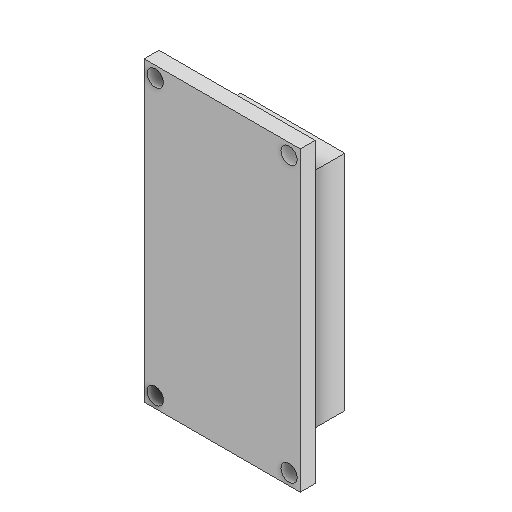
# Autodesk Inventor part: 7_Seg_Display_TM1637
Saved by Autodesk Inventor 2026.2 (Build 302298010, 298A)
## iProperties
Created: 2026-03-17
Part Number: 7_Seg_Display_TM1637
Material: Generic
Document SubType Name: Modeling
Designer: vckot
Density: 1 g/cm^3
Appearance: Default
Author: vckot
Autodesk Inventor part; units mm, degrees
ref_plane "YZ Plane" through (0, 0, 0) normal (1, 0, 0) x (0, 1, 0)
ref_plane "XZ Plane" through (0, 0, 0) normal (0, 1, 0) x (-1, 0, 0)
ref_plane "XY Plane" through (0, 0, 0) normal (0, 0, 1) x (1, 0, 0)
sketch "Sketch1" plane through (0, 0, 0) normal (0, 1, 0) x (-1, 0, 0)
  line L0 (-10.5, 20) -> (10.5, 20)
  line L1 (10.5, 20) -> (10.5, -20)
  line L2 (10.5, -20) -> (-10.5, -20)
  line L3 (-10.5, -20) -> (-10.5, 20)
  line L4 (-10.5, 20) -> (10.5, -20) construction
  line L5 (10.5, 20) -> (-10.5, -20) construction
  point P0 (0, 0)
  dimension "d0" = 40
  dimension "d1" = 21
  constraints: 12 end point, 2 midpoint, 2 parallel, 1 horizontal, 1 perpendicular
  measures "d0" distance of L0.end L1.end
  measures "d1" distance of L1.end L2.end
extrude "Extrusion1" add sketch "Sketch1" along normal blind 2
sketch "Sketch2" plane through (0, 2, 0) normal (0, 1, 0) x (1, 0, 0)
  line L0 (-10.5, 20) -> (-10.5, -20) projected
  line L1 (-10.5, -20) -> (10.5, -20) projected
  line L2 (10.5, -20) -> (10.5, 20) projected
  line L3 (10.5, 20) -> (-10.5, 20) projected
  point P0 (0, 0)
  point P1 (-9, -18.5)
  point P2 (-9, 18.5)
  point P3 (9, 18.5)
  point P4 (9, -18.5)
  dimension "d4" = 1.5
  dimension "d5" = 1.5
  dimension "d6" = 1.5
  dimension "d7" = 1.5
  dimension "d20" = 18
  dimension "d21" = 18
  dimension "d22" = 37
  constraints: 2 horizontal alignment, 2 vertical alignment
  measures "d4" distance from line of L0 point (-9, -18.5)
  measures "d5" distance from line of L1 point (-9, -18.5)
  measures "d6" distance from line of L2 point (9, -18.5)
  measures "d7" distance from line of L3 point (-9, 18.5)
  measures "d20" distance of point (9, 18.5) point (-9, 18.5)
  measures "d21" distance of point (9, -18.5) point (-9, -18.5)
  measures "d22" distance of point (-9, 18.5) point (-9, -18.5)
hole "Hole1" at (-9, 2, 18.5) at (-9, 2, -18.5) at (9, 2, -18.5) at (9, 2, 18.5) direction (0, -1, 0) diameter 2.2 end through all
sketch "Sketch3" plane through (0, 2, 0) normal (0, 1, 0) x (1, 0, 0)
  line L0 (7.5, -13.5) -> (-6.5, -13.5)
  line L1 (-6.5, -13.5) -> (-6.5, 16.5)
  line L2 (-6.5, 16.5) -> (7.5, 16.5)
  line L3 (7.5, 16.5) -> (7.5, -13.5)
  line L4 (7.5, -13.5) -> (-6.5, 16.5) construction
  line L5 (-6.5, -13.5) -> (7.5, 16.5) construction
  line L6 (-10.5, -20) -> (10.5, -20) projected
  line L7 (-10.5, 20) -> (-10.5, -20) projected
  line L8 (10.5, 20) -> (-10.5, 20) projected
  point P0 (0, 0)
  point P1 (0.5, 1.5)
  point P2 (0, -20)
  dimension "d15" = 6.5
  dimension "d16" = 30
  dimension "d17" = 14
  dimension "d18" = 4
  dimension "d19" = 3.5
  constraints: 12 end point, 3 midpoint, 2 parallel, 1 horizontal, 1 perpendicular
  measures "d15" distance from line of point (0, -20) L0
  measures "d16" distance of L0.end L1.end
  measures "d17" distance of L1.end L2.end
  measures "d18" distance between parallel lines of L7 L1
  measures "d19" distance between parallel lines of L8 L2
extrude "Extrusion2" add sketch "Sketch3" along normal blind 7
sketch "Sketch4" plane through (0, 9, 0) normal (0, 1, 0) x (1, 0, 0)
  line L0 (-6.5, -13.5) -> (7.5, -13.5) projected
  line L1 (10.5, -20) -> (10.5, 20) projected
  line L2 (-6.5, 16.5) -> (-6.5, -13.5) projected
  line L3 (-0.449, -7.3714) -> (-0.0305, -6.9347)
  line L4 (-0.0305, -6.9347) -> (0.3941, -7.3714)
  line L5 (0.3941, -7.3714) -> (0.3941, -10.3494)
  line L6 (0.3941, -10.3494) -> (-0.0305, -10.774)
  line L7 (-0.0305, -10.774) -> (-0.449, -10.3494)
  line L8 (-0.449, -10.3494) -> (-0.449, -7.3714)
  line L9 (-0.5096, -11.2532) -> (-4.0275, -11.2532)
  line L10 (-4.0275, -11.2532) -> (-3.1723, -10.398)
  line L11 (-3.1723, -10.398) -> (-0.728, -10.398)
  line L12 (-0.728, -10.398) -> (-0.1882, -10.9317)
  line L13 (-0.1882, -10.9317) -> (-0.5096, -11.2532)
  line L14 (0.6731, -10.398) -> (3.1174, -10.398)
  line L15 (3.1174, -10.398) -> (3.9725, -11.2532)
  line L16 (3.9725, -11.2532) -> (0.4669, -11.2532)
  line L17 (0.4669, -11.2532) -> (0.1333, -10.9317)
  line L18 (0.1333, -10.9317) -> (0.6731, -10.398)
  line L19 (-0.7219, -7.3108) -> (-3.1662, -7.3108)
  line L20 (-3.1662, -7.3108) -> (-4.0275, -6.4677)
  line L21 (-4.0275, -6.4677) -> (-0.5036, -6.4677)
  line L22 (-0.5036, -6.4677) -> (-0.1882, -6.777)
  line L23 (-0.1882, -6.777) -> (-0.7219, -7.3108)
  line L24 (0.4669, -6.4677) -> (3.9725, -6.4677)
  line L25 (3.9725, -6.4677) -> (3.1174, -7.3108)
  line L26 (3.1174, -7.3108) -> (0.6731, -7.3108)
  line L27 (0.6731, -7.3108) -> (0.1333, -6.777)
  line L28 (0.1333, -6.777) -> (0.4669, -6.4677)
  line L29 (-0.449, -1.2092) -> (-0.0305, -0.7725)
  line L30 (-0.0305, -0.7725) -> (0.3941, -1.2092)
  line L31 (0.3941, -1.2092) -> (0.3941, -4.1872)
  line L32 (0.3941, -4.1872) -> (-0.0305, -4.6118)
  line L33 (-0.0305, -4.6118) -> (-0.449, -4.1872)
  line L34 (-0.449, -4.1872) -> (-0.449, -1.2092)
  line L35 (-0.5096, -5.0909) -> (-4.0275, -5.0909)
  line L36 (-4.0275, -5.0909) -> (-3.1723, -4.2357)
  line L37 (-3.1723, -4.2357) -> (-0.728, -4.2357)
  line L38 (-0.728, -4.2357) -> (-0.1882, -4.7695)
  line L39 (-0.1882, -4.7695) -> (-0.5096, -5.0909)
  line L40 (0.6731, -4.2357) -> (3.1174, -4.2357)
  line L41 (3.1174, -4.2357) -> (3.9725, -5.0909)
  line L42 (3.9725, -5.0909) -> (0.4669, -5.0909)
  line L43 (0.4669, -5.0909) -> (0.1333, -4.7695)
  line L44 (0.1333, -4.7695) -> (0.6731, -4.2357)
  line L45 (-0.7219, -1.1485) -> (-3.1662, -1.1485)
  line L46 (-3.1662, -1.1485) -> (-4.0275, -0.3055)
  line L47 (-4.0275, -0.3055) -> (-0.5036, -0.3055)
  line L48 (-0.5036, -0.3055) -> (-0.1882, -0.6148)
  line L49 (-0.1882, -0.6148) -> (-0.7219, -1.1485)
  line L50 (0.4669, -0.3055) -> (3.9725, -0.3055)
  line L51 (3.9725, -0.3055) -> (3.1174, -1.1485)
  line L52 (3.1174, -1.1485) -> (0.6731, -1.1485)
  line L53 (0.6731, -1.1485) -> (0.1333, -0.6148)
  line L54 (0.1333, -0.6148) -> (0.4669, -0.3055)
  line L55 (-1.8319, 1.3321) -> (-2.687, 1.3321)
  line L56 (-2.687, 1.3321) -> (-2.687, 2.1873)
  line L57 (-2.687, 2.1873) -> (-1.8319, 2.1873)
  line L58 (-1.8319, 2.1873) -> (-1.8319, 1.3321)
  line L59 (3.9725, 1.3321) -> (3.1174, 1.3321)
  line L60 (3.1174, 1.3321) -> (3.1174, 2.1873)
  line L61 (3.1174, 2.1873) -> (3.9725, 2.1873)
  line L62 (3.9725, 2.1873) -> (3.9725, 1.3321)
  line L63 (-4.0275, 8.4527) -> (-3.1723, 7.6035)
  line L64 (-3.1723, 7.6035) -> (-3.1723, 4.8257)
  line L65 (-3.1723, 4.8257) -> (-4.0275, 3.9826)
  line L66 (-4.0275, 3.9826) -> (-4.0275, 8.4527)
  line L67 (0.6731, 4.6801) -> (3.1174, 4.6801)
  line L68 (3.1174, 4.6801) -> (3.9725, 3.8249)
  line L69 (3.9725, 3.8249) -> (0.4669, 3.8249)
  line L70 (0.4669, 3.8249) -> (0.1333, 4.1464)
  line L71 (0.1333, 4.1464) -> (0.6731, 4.6801)
  line L72 (0.4669, 8.6104) -> (3.9725, 8.6104)
  line L73 (3.9725, 8.6104) -> (3.1174, 7.7673)
  line L74 (3.1174, 7.7673) -> (0.6731, 7.7673)
  line L75 (0.6731, 7.7673) -> (0.1333, 8.301)
  line L76 (0.1333, 8.301) -> (0.4669, 8.6104)
  line L77 (-0.5096, 3.8249) -> (-3.8698, 3.8249)
  line L78 (-3.8698, 3.8249) -> (-3.0085, 4.6801)
  line L79 (-3.0085, 4.6801) -> (-0.728, 4.6801)
  line L80 (-0.728, 4.6801) -> (-0.1882, 4.1464)
  line L81 (-0.1882, 4.1464) -> (-0.5096, 3.8249)
  line L82 (-0.7219, 7.7673) -> (-3.0085, 7.7673)
  line L83 (-3.0085, 7.7673) -> (-3.8637, 8.6104)
  line L84 (-3.8637, 8.6104) -> (-0.5036, 8.6104)
  line L85 (-0.5036, 8.6104) -> (-0.1882, 8.301)
  line L86 (-0.1882, 8.301) -> (-0.7219, 7.7673)
  line L87 (-2.5294, 5.7901) -> (-2.9539, 6.2146)
  line L88 (-2.9539, 6.2146) -> (-2.5294, 6.6452)
  line L89 (-2.5294, 6.6452) -> (-0.6249, 6.6452)
  line L90 (-0.6249, 6.6452) -> (-0.1882, 6.2146)
  line L91 (-0.1882, 6.2146) -> (-0.6249, 5.7901)
  line L92 (-0.6249, 5.7901) -> (-2.5294, 5.7901)
  line L93 (-4.0275, 14.6149) -> (-3.1723, 13.7658)
  line L94 (-3.1723, 13.7658) -> (-3.1723, 10.9879)
  line L95 (-3.1723, 10.9879) -> (-4.0275, 10.1449)
  line L96 (-4.0275, 10.1449) -> (-4.0275, 14.6149)
  line L97 (0.6731, 10.8424) -> (3.1174, 10.8424)
  line L98 (3.1174, 10.8424) -> (3.9725, 9.9872)
  line L99 (3.9725, 9.9872) -> (0.4669, 9.9872)
  line L100 (0.4669, 9.9872) -> (0.1333, 10.3086)
  line L101 (0.1333, 10.3086) -> (0.6731, 10.8424)
  line L102 (0.4669, 14.7726) -> (3.9725, 14.7726)
  line L103 (3.9725, 14.7726) -> (3.1174, 13.9296)
  line L104 (3.1174, 13.9296) -> (0.6731, 13.9296)
  line L105 (0.6731, 13.9296) -> (0.1333, 14.4633)
  line L106 (0.1333, 14.4633) -> (0.4669, 14.7726)
  line L107 (-0.5096, 9.9872) -> (-3.8698, 9.9872)
  line L108 (-3.8698, 9.9872) -> (-3.0085, 10.8424)
  line L109 (-3.0085, 10.8424) -> (-0.728, 10.8424)
  line L110 (-0.728, 10.8424) -> (-0.1882, 10.3086)
  line L111 (-0.1882, 10.3086) -> (-0.5096, 9.9872)
  line L112 (-0.7219, 13.9296) -> (-3.0085, 13.9296)
  line L113 (-3.0085, 13.9296) -> (-3.8637, 14.7726)
  line L114 (-3.8637, 14.7726) -> (-0.5036, 14.7726)
  line L115 (-0.5036, 14.7726) -> (-0.1882, 14.4633)
  line L116 (-0.1882, 14.4633) -> (-0.7219, 13.9296)
  line L117 (-2.5294, 11.9523) -> (-2.9539, 12.3769)
  line L118 (-2.9539, 12.3769) -> (-2.5294, 12.8075)
  line L119 (-2.5294, 12.8075) -> (-0.6249, 12.8075)
  line L120 (-0.6249, 12.8075) -> (-0.1882, 12.3769)
  line L121 (-0.1882, 12.3769) -> (-0.6249, 11.9523)
  line L122 (-0.6249, 11.9523) -> (-2.5294, 11.9523)
  point P0 (0, 0)
  point P1 (-4.0275, -11.9385)
  constraints: 1 other
extrude "Extrusion3" add sketch "Sketch4" along normal blind 0.1
body "Solid1"
